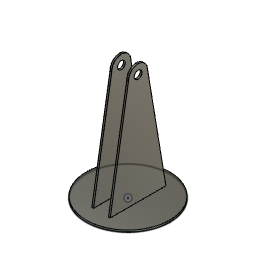
base v1 (Autodesk Fusion 360 design; units mm, degrees)
Autodesk Fusion 360 part; units mm, degrees
sketch "Sketch1" plane through (0, 0, 0) normal (0, 0, 1) x (1, 0, 0)
  circle A0 centre (0, 0) radius 150
  dimension "d1" = 300
  constraint coincident A0.centre origin
  measures "d1" diameter of A0
extrude "Extrude1" add sketch "Sketch1" along normal blind 6.2 makes body 1
sketch "Sketch3" plane through (0, 0, 0) normal (1, 0, 0) x (0, 1, 0)
  line L0 (0, 6.2) -> (100, 6.2)
  line L1 (0, 6.2) -> (0, 436.2) construction
  circle A0 centre (0, 402.2) radius 14
  line L2 (0, 402.2) -> (-14, 402.2) construction
  line L3 (0, 402.2) -> (14, 402.2) construction
  line L4 (14, 402.2) -> (34, 402.2) construction
  line L5 (34.6123, 398.526) -> (100, 6.2)
  arc A1 (33.9262, 404.4389) -> (0, 436.2) centre (0, 402.2) ccw
  line L6 (-14, 402.2) -> (-34, 402.2) construction
  arc A2 (33.9262, 404.4389) -> (34.6123, 398.526) centre (93.796, 408.3899) ccw
  arc A3 (0, 436.2) -> (-33.9262, 404.4389) centre (0, 402.2) ccw
  line L7 (-34.6123, 398.526) -> (-100, 6.2)
  line L8 (0, 6.2) -> (-100, 6.2)
  arc A4 (-34.6123, 398.526) -> (-33.9262, 404.4389) centre (-93.796, 408.3899) ccw
  point P0 (0, 6.2)
  dimension "d11" = 430
  dimension "d13" = 28
  dimension "d14" = 20
  dimension "d15" = 60
  constraint horizontal L0
  constraint perpendicular L0 L1
  constraint concentric A0 A1
  constraint coincident A0.centre L2.start
  constraint coincident A0 L2.end
  constraint perpendicular L1 L2
  constraint coincident A0 L3.end
  constraint perpendicular L1 L3
  constraint parallel L3 L4
  constraint parallel L2 L6
  constraint coincident L4.end L5
  constraint coincident L4.end A1
  constraint tangent L5 A2
  constraint tangent A1 A2
  constraint symmetric P0 L1 L0.start
  constraint symmetric L0.end L1 L7.end
  constraint symmetric A1.end L1 A3.start
  constraint symmetric L1 A1 A3
  constraint symmetric L1 L5.start L7.start
  constraint symmetric L1 A1.start A3.end
  constraint symmetric L1 A2 A4
  constraint coincident P0 L0.start
  measures "d11" distance of P0 L1.end
  measures "d13" diameter of A0
  measures "d14" distance of A0 A1
  measures "d15" radius of A2
extrude "Extrude2" add sketch "Sketch3" along normal blind 6.2 separate body makes body 2
copy_body "CopyPasteBodies1" bodies 2 makes body 3
move_body "Move1" bodies 3 to x (1, 0, 0) y (0, 1, 0) z (0, 0, 1) at (30, 0, 0)
move_body "Move2" bodies 2 to x (1, 0, 0) y (0, 1, 0) z (0, 0, 1) at (-30, 0, 0)
